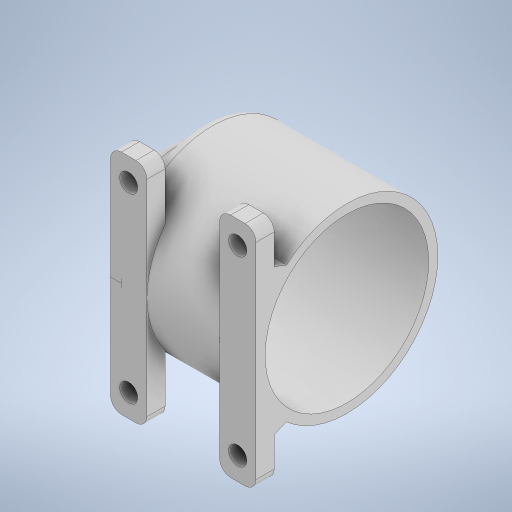
# Autodesk Inventor part: Motor
Saved by Autodesk Inventor 2023 (Build 270158000, 158)
## iProperties
Created: 2023-07-24
Part Number: Motor
Material: Generic
Document SubType Name: Modeling
Designer: User
Density: 1 g/cm^3
Appearance: Default
Author: User
Autodesk Inventor part; units mm, degrees
ref_plane "YZ Plane" through (0, 0, 0) normal (1, 0, 0) x (0, 1, 0)
ref_plane "XZ Plane" through (0, 0, 0) normal (0, 1, 0) x (-1, 0, 0)
sketch "Sketch1" plane through (0, 0, 0) normal (0, 0, 1) x (1, 0, 0)
  line L0 (0, 0) -> (22.5769, 0) construction
  line L1 (0, 10) -> (0, 24)
  line L2 (6, 30) -> (14, 30)
  line L3 (20, 36) -> (20, 50)
  line L4 (20, 50) -> (100, 50)
  arc A0 (6, 30) -> (0, 24) centre (6, 24) ccw
  arc A1 (14, 30) -> (20, 36) centre (14, 36) ccw
  line L5 (100, 45) -> (25, 45)
  line L6 (25, 45) -> (25, 36)
  arc A2 (14, 25) -> (25, 36) centre (14, 36) ccw
  line L7 (14, 25) -> (6, 25)
  arc A3 (6, 25) -> (5, 24) centre (6, 24) ccw
  line L8 (5, 24) -> (5, 10)
  line L9 (100, 50) -> (100, 45)
  line L10 (5, 10) -> (0, 10)
  point P0 (20, 30)
  point P1 (0, 17)
  point P2 (20, 43)
  dimension "d0" = 10
  dimension "d1" = 20
  dimension "d2" = 80
  dimension "d3" = 30
  dimension "d4" = 50
  dimension "d5" = 6
  dimension "d6" = 5
  constraints: 22 end point, 8 point on circle, 6 perpendicular, 4 centre point, 4 tangent, 2 horizontal, 2 midpoint, 2 point on line, 2 vertical, 1 equal radius, 5 other
  measures "d0" distance from line of L0 L1.start
  measures "d1" horizontal distance of point (20, 30) point (0, 17)
  measures "d2" horizontal distance of L4.end point (20, 43)
  measures "d3" distance between parallel lines of L2 L0
  measures "d4" distance between parallel lines of L4 L0
  measures "d5" radius of A0
  measures "d6" distance between parallel lines of L4 L5
revolve "Revolution1" add sketch "Sketch1" angle 360 about axis through (0, 0, 0) along (1, 0, 0)
fillet "Fillet1" radius 6 1 edges at (20, -50, 0)
sketch "Sketch2" plane through (100, 0, 0) normal (1, 0, 0) x (0, 0, -1)
  line L0 (-40, 62.5) -> (-50, 62.5)
  line L1 (-50, 62.5) -> (-50, -62.5)
  line L2 (-50, -62.5) -> (-40, -62.5)
  circle A0 centre (0, 0) radius 50 projected
  line L3 (-40, -62.5) -> (-40, -30)
  line L4 (-40, 30) -> (-40, 62.5)
  point P0 (-45, -62.5)
  point P1 (-50, 0)
  dimension "d9" = 10
  dimension "d10" = 125
  dimension "d11" = 62.5
  constraints: 10 end point, 3 parallel, 2 point on circle, 1 horizontal, 1 midpoint, 1 perpendicular, 1 tangent
  measures "d9" distance of L1.end L2.end
  measures "d10" distance of L0.end L1.end
  measures "d11" vertical distance of point (0, 0) point (-45, -62.5)
extrude "Extrusion1" add sketch "Sketch2" against normal blind 20 contours L4 A0 L1 L0 | A0 L3 L2 L1
chamfer "Chamfer1" distance 10 angle 45 2 edges at (90, -30, 40) (90, 30, 40)
fillet "Fillet3" radius 6 4 edges at (100, 62.5, 45) (100, -62.5, 45) (80, -62.5, 45) (80, 62.5, 45)
sketch "Sketch3" plane through (100, -40, 40) normal (0, 0, -1) x (-1, 0, 0)
  line L0 (20, 0) -> (20, -16.5) projected
  line L1 (0, 0) -> (20, 0) projected
  line L2 (20, 96.5) -> (20, 80) projected
  line L3 (20, 80) -> (0, 80) projected
  point P0 (100, 40)
  point P1 (10, -10)
  point P2 (10, 90)
  dimension "d19" = 10
  dimension "d20" = 10
  dimension "d21" = 10
  dimension "d22" = 10
  measures "d19" distance from line of L0 point (10, -10)
  measures "d20" distance from line of L1 point (10, -10)
  measures "d21" distance from line of L2 point (10, 90)
  measures "d22" distance from line of L3 point (10, 90)
hole "Hole1" at (90, -50, 40) at (90, 50, 40) direction (0, 0, 1) diameter 10 end through all
ref_plane "Work Plane1" through (60, 0, 0) normal (-1, 0, 0) x (0, 0, 1)
mirror "Mirror1" about plane through (60, 0, 0) normal (-1, 0, 0) of "Hole1", "Extrusion1", "Fillet3"
body "Solid1"
